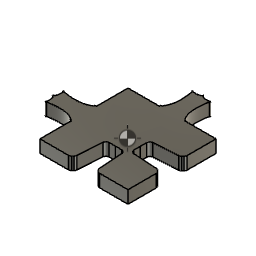
peg-design-block v3 (Autodesk Fusion 360 design; units mm, degrees)
Autodesk Fusion 360 part; units mm, degrees
note: some values were not read from the file. Set by a fixed rule: which sketch regions a step uses.
sketch "Sketch1" plane through (0, 0, 0) normal (0, 0, 1) x (1, 0, 0)
  line L0 (10, 10) -> (-10, 10)
  line L1 (0, 10) -> (0, 20)
  line L2 (-10, 10) -> (-4, 10)
  line L3 (10, 10) -> (4, 10)
  line L4 (0, 20) -> (0, 19.3)
  line L5 (0, 20) -> (0, 19.9)
  line L6 (-3, 11) -> (-2.5, 11)
  line L7 (3, 11) -> (2.5, 11)
  line L8 (-10, 10) -> (-11, 10)
  line L9 (11, 10) -> (10, 10)
  line L10 (0, 10) -> (-4.5, 10)
  line L11 (0, 10) -> (4.5, 10)
  line L12 (0, 10) -> (0, 20)
  line L13 (4, 10.5) -> (4, 10.4)
  line L14 (4, 10.5) -> (4, 10.4)
  line L15 (-2.5, 11) -> (-2.5, 13.5)
  line L16 (2.5, 11) -> (2.5, 13.5)
  line L17 (-4, 10) -> (-3.8, 10)
  line L18 (-4, 10) -> (-3.8, 10.3)
  circle A0 centre (-3.8, 10.3) radius 0.2
  circle A1 centre (3.8, 10.3) radius 0.2
  line L19 (3.8, 10.3) -> (4, 10)
  line L20 (0, 20) -> (0, 19.4)
  line L21 (0, 20) -> (0, 19.3)
  circle A2 centre (2.8, 19.3) radius 0.2
  circle A3 centre (-2.8, 19.3) radius 0.2
  line L22 (0, 20) -> (0, 19.8)
  circle A4 centre (0, 19.8) radius 0.2
  spline S0 degree 5 poles (0, 19.8) (-0.0322, 19.7692) (-0.0986, 19.7096) (-0.2048, 19.6258) (-0.3594, 19.5254) (-0.576, 19.4201) (-0.8177, 19.3367) (-1.0861, 19.2766) (-1.3815, 19.2401) (-1.7022, 19.2255) (-2.046, 19.2311) (-2.3378, 19.2501) (-2.5655, 19.2721) (-2.7212, 19.2901) (-2.8, 19.3) knots 0 0 0 0 0 0 0.1 0.2 0.3 0.4 0.5 0.6 0.7 0.8 0.9 1 1 1 1 1 1
  spline S1 degree 5 poles (0, 19.8) (0.0322, 19.7692) (0.0986, 19.7096) (0.2048, 19.6258) (0.3594, 19.5254) (0.576, 19.4201) (0.8177, 19.3367) (1.0861, 19.2766) (1.3815, 19.2401) (1.7022, 19.2255) (2.046, 19.2311) (2.3378, 19.2501) (2.5655, 19.2721) (2.7212, 19.2901) (2.8, 19.3) knots 0 0 0 0 0 0 0.1 0.2 0.3 0.4 0.5 0.6 0.7 0.8 0.9 1 1 1 1 1 1
  spline S2 degree 5 poles (-2.8, 19.3) (-2.7571, 19.0585) (-2.6765, 18.5805) (-2.5713, 17.879) (-2.4629, 16.9749) (-2.3846, 15.9005) (-2.3693, 14.8878) (-2.4235, 13.943) (-2.5527, 13.0716) (-2.7578, 12.2743) (-3.0346, 11.5472) (-3.3095, 11.0177) (-3.5439, 10.6483) (-3.7126, 10.4141) (-3.8, 10.3) knots 0 0 0 0 0 0 0.1 0.2 0.3 0.4 0.5 0.6 0.7 0.8 0.9 1 1 1 1 1 1
  spline S3 degree 5 poles (2.8, 19.3) (2.7571, 19.0585) (2.6765, 18.5805) (2.5713, 17.879) (2.4629, 16.9749) (2.3846, 15.9005) (2.3693, 14.8878) (2.4235, 13.943) (2.5527, 13.0716) (2.7578, 12.2743) (3.0346, 11.5472) (3.3095, 11.0177) (3.5439, 10.6483) (3.7126, 10.4141) (3.8, 10.3) knots 0 0 0 0 0 0 0.1 0.2 0.3 0.4 0.5 0.6 0.7 0.8 0.9 1 1 1 1 1 1
  line L23 (-2.8, 19.3) -> (-2.8, 19.5)
  line L24 (-2.8, 19.5) -> (-3, 19.5)
  line L25 (0, 20) -> (0, 19.8)
  line L26 (0, 20) -> (0, 19.3)
  line L27 (0, 20) -> (0, 19.9)
  circle A5 centre (0, 19.8) radius 0.2
  line L28 (0, 10) -> (0, 20)
  line L29 (4, 10.5) -> (4, 10.4)
  line L30 (0, 10) -> (0, 20)
  line L31 (4, 10.5) -> (4, 10.4)
  circle A6 centre (3.8, 10.3) radius 0.2
  line L32 (-4, 10) -> (-3.8, 10)
  line L33 (3.8, 10.3) -> (4, 10)
  line L34 (3, 11) -> (2.5, 11)
  line L35 (-3, 11) -> (-2.5, 11)
  circle A7 centre (-3.8, 10.3) radius 0.2
  line L36 (-4, 10) -> (-3.8, 10.3)
  line L37 (4, 10) -> (4, 10.5)
  circle A8 centre (-2.8, 19.3) radius 0.2
  line L38 (-2.8, 19.5) -> (-3, 19.5)
  line L39 (2.5, 11) -> (2.5, 13.5)
  line L40 (0, 10) -> (-4.5, 10)
  line L41 (-2.5, 11) -> (-2.5, 13.5)
  line L42 (0, 20) -> (0, 19.3)
  spline S4 degree 5 poles (-2.8, 19.3) (-2.7571, 19.0585) (-2.6765, 18.5805) (-2.5713, 17.879) (-2.4629, 16.9749) (-2.3846, 15.9005) (-2.3693, 14.8878) (-2.4235, 13.943) (-2.5527, 13.0716) (-2.7578, 12.2743) (-3.0346, 11.5472) (-3.3095, 11.0177) (-3.5439, 10.6483) (-3.7126, 10.4141) (-3.8, 10.3) knots 0 0 0 0 0 0 0.1 0.2 0.3 0.4 0.5 0.6 0.7 0.8 0.9 1 1 1 1 1 1
  line L43 (0, 20) -> (0, 19.4)
  spline S5 degree 5 poles (0, 19.8) (-0.0322, 19.7692) (-0.0986, 19.7096) (-0.2048, 19.6258) (-0.3594, 19.5254) (-0.576, 19.4201) (-0.8177, 19.3367) (-1.0861, 19.2766) (-1.3815, 19.2401) (-1.7022, 19.2255) (-2.046, 19.2311) (-2.3378, 19.2501) (-2.5655, 19.2721) (-2.7212, 19.2901) (-2.8, 19.3) knots 0 0 0 0 0 0 0.1 0.2 0.3 0.4 0.5 0.6 0.7 0.8 0.9 1 1 1 1 1 1
  circle A9 centre (2.8, 19.3) radius 0.2
  spline S6 degree 5 poles (0, 19.8) (0.0322, 19.7692) (0.0986, 19.7096) (0.2048, 19.6258) (0.3594, 19.5254) (0.576, 19.4201) (0.8177, 19.3367) (1.0861, 19.2766) (1.3815, 19.2401) (1.7022, 19.2255) (2.046, 19.2311) (2.3378, 19.2501) (2.5655, 19.2721) (2.7212, 19.2901) (2.8, 19.3) knots 0 0 0 0 0 0 0.1 0.2 0.3 0.4 0.5 0.6 0.7 0.8 0.9 1 1 1 1 1 1
  line L44 (-2.8, 19.3) -> (-2.8, 19.5)
  spline S7 degree 5 poles (2.8, 19.3) (2.7571, 19.0585) (2.6765, 18.5805) (2.5713, 17.879) (2.4629, 16.9749) (2.3846, 15.9005) (2.3693, 14.8878) (2.4235, 13.943) (2.5527, 13.0716) (2.7578, 12.2743) (3.0346, 11.5472) (3.3095, 11.0177) (3.5439, 10.6483) (3.7126, 10.4141) (3.8, 10.3) knots 0 0 0 0 0 0 0.1 0.2 0.3 0.4 0.5 0.6 0.7 0.8 0.9 1 1 1 1 1 1
  line L45 (0, 20) -> (0, 19.8)
  line L46 (0, 20) -> (0, 19.3)
  line L47 (0, 20) -> (0, 19.9)
  circle A10 centre (0, 19.8) radius 0.2
  line L48 (0, 10) -> (0, 20)
  line L49 (4, 10.5) -> (4, 10.4)
  line L50 (0, 10) -> (0, 20)
  line L51 (4, 10.5) -> (4, 10.4)
  circle A11 centre (3.8, 10.3) radius 0.2
  line L52 (-4, 10) -> (-3.8, 10)
  line L53 (3.8, 10.3) -> (4, 10)
  line L54 (3, 11) -> (2.5, 11)
  line L55 (-3, 11) -> (-2.5, 11)
  circle A12 centre (-3.8, 10.3) radius 0.2
  line L56 (-4, 10) -> (-3.8, 10.3)
  circle A13 centre (-2.8, 19.3) radius 0.2
  line L57 (-2.8, 19.5) -> (-3, 19.5)
  line L58 (2.5, 11) -> (2.5, 13.5)
  line L59 (0, 10) -> (-4.5, 10)
  line L60 (-2.5, 11) -> (-2.5, 13.5)
  line L61 (0, 20) -> (0, 19.3)
  spline S8 degree 5 poles (-2.8, 19.3) (-2.7571, 19.0585) (-2.6765, 18.5805) (-2.5713, 17.879) (-2.4629, 16.9749) (-2.3846, 15.9005) (-2.3693, 14.8878) (-2.4235, 13.943) (-2.5527, 13.0716) (-2.7578, 12.2743) (-3.0346, 11.5472) (-3.3095, 11.0177) (-3.5439, 10.6483) (-3.7126, 10.4141) (-3.8, 10.3) knots 0 0 0 0 0 0 0.1 0.2 0.3 0.4 0.5 0.6 0.7 0.8 0.9 1 1 1 1 1 1
  line L62 (0, 20) -> (0, 19.4)
  spline S9 degree 5 poles (0, 19.8) (-0.0322, 19.7692) (-0.0986, 19.7096) (-0.2048, 19.6258) (-0.3594, 19.5254) (-0.576, 19.4201) (-0.8177, 19.3367) (-1.0861, 19.2766) (-1.3815, 19.2401) (-1.7022, 19.2255) (-2.046, 19.2311) (-2.3378, 19.2501) (-2.5655, 19.2721) (-2.7212, 19.2901) (-2.8, 19.3) knots 0 0 0 0 0 0 0.1 0.2 0.3 0.4 0.5 0.6 0.7 0.8 0.9 1 1 1 1 1 1
  circle A14 centre (2.8, 19.3) radius 0.2
  spline S10 degree 5 poles (0, 19.8) (0.0322, 19.7692) (0.0986, 19.7096) (0.2048, 19.6258) (0.3594, 19.5254) (0.576, 19.4201) (0.8177, 19.3367) (1.0861, 19.2766) (1.3815, 19.2401) (1.7022, 19.2255) (2.046, 19.2311) (2.3378, 19.2501) (2.5655, 19.2721) (2.7212, 19.2901) (2.8, 19.3) knots 0 0 0 0 0 0 0.1 0.2 0.3 0.4 0.5 0.6 0.7 0.8 0.9 1 1 1 1 1 1
  line L63 (-2.8, 19.3) -> (-2.8, 19.5)
  spline S11 degree 5 poles (2.8, 19.3) (2.7571, 19.0585) (2.6765, 18.5805) (2.5713, 17.879) (2.4629, 16.9749) (2.3846, 15.9005) (2.3693, 14.8878) (2.4235, 13.943) (2.5527, 13.0716) (2.7578, 12.2743) (3.0346, 11.5472) (3.3095, 11.0177) (3.5439, 10.6483) (3.7126, 10.4141) (3.8, 10.3) knots 0 0 0 0 0 0 0.1 0.2 0.3 0.4 0.5 0.6 0.7 0.8 0.9 1 1 1 1 1 1
  line L64 (-11, 10) -> (-12, 10)
  line L65 (12, 10) -> (11, 10)
  line L66 (-12, 10) -> (-14, 10)
  line L67 (-14, 10) -> (-14, -18)
  line L68 (-14, -18) -> (14, -18)
  line L69 (14, -18) -> (14, 10)
  line L70 (14, 10) -> (12, 10)
  line L71 (-14, 10) -> (14, -18)
  line L72 (-2.9666, -8.002) -> (0, -8)
  line L73 (2.9666, -8.002) -> (0, -8)
  line L74 (-3, -8.5) -> (-2.9666, -8.002)
  line L75 (3, -8.5) -> (2.9666, -8.002)
  line L76 (-3.5757, -17.0757) -> (-3, -8.5)
  line L77 (3.5757, -17.0757) -> (3, -8.5)
  line L78 (-4, -17.5) -> (-3.5757, -17.0757)
  line L79 (4, -17.5) -> (3.5757, -17.0757)
  line L80 (-4.5, -18) -> (-4, -17.5)
  line L81 (4.5, -18) -> (4, -17.5)
  line L82 (4.002, -7.0666) -> (4, -4.1)
  line L83 (4.002, -1.1334) -> (4, -4.1)
  line L84 (4.5, -7.1) -> (4.002, -7.0666)
  line L85 (4.5, -1.1) -> (4.002, -1.1334)
  line L86 (13.0757, -7.6757) -> (4.5, -7.1)
  line L87 (13.0757, -0.5243) -> (4.5, -1.1)
  line L88 (13.5, -8.1) -> (13.0757, -7.6757)
  line L89 (13.5, -0.1) -> (13.0757, -0.5243)
  line L90 (14, -8.6) -> (13.5, -8.1)
  line L91 (14, 0.4) -> (13.5, -0.1)
  line L92 (-14.5, 0) -> (-14.4, 0)
  line L93 (-15, -1.5) -> (-17.5, -1.5)
  line L94 (-14.3, -0.2) -> (-14, 0)
  line L95 (-14.5, 0) -> (-14.4, 0)
  line L96 (-14, -4) -> (-14, -8.5)
  line L97 (-23.5, -6.8) -> (-23.5, -7)
  spline S12 degree 5 poles (-23.3, -6.8) (-23.0585, -6.7571) (-22.5805, -6.6765) (-21.879, -6.5713) (-20.9749, -6.4629) (-19.9005, -6.3846) (-18.8878, -6.3693) (-17.943, -6.4235) (-17.0716, -6.5527) (-16.2743, -6.7578) (-15.5472, -7.0346) (-15.0177, -7.3095) (-14.6483, -7.5439) (-14.4141, -7.7126) (-14.3, -7.8) knots 0 0 0 0 0 0 0.1 0.2 0.3 0.4 0.5 0.6 0.7 0.8 0.9 1 1 1 1 1 1
  spline S13 degree 5 poles (-23.3, -6.8) (-23.0585, -6.7571) (-22.5805, -6.6765) (-21.879, -6.5713) (-20.9749, -6.4629) (-19.9005, -6.3846) (-18.8878, -6.3693) (-17.943, -6.4235) (-17.0716, -6.5527) (-16.2743, -6.7578) (-15.5472, -7.0346) (-15.0177, -7.3095) (-14.6483, -7.5439) (-14.4141, -7.7126) (-14.3, -7.8) knots 0 0 0 0 0 0 0.1 0.2 0.3 0.4 0.5 0.6 0.7 0.8 0.9 1 1 1 1 1 1
  spline S14 degree 5 poles (-23.3, -1.2) (-23.0585, -1.2429) (-22.5805, -1.3235) (-21.879, -1.4287) (-20.9749, -1.5371) (-19.9005, -1.6154) (-18.8878, -1.6307) (-17.943, -1.5765) (-17.0716, -1.4473) (-16.2743, -1.2422) (-15.5472, -0.9654) (-15.0177, -0.6905) (-14.6483, -0.4561) (-14.4141, -0.2874) (-14.3, -0.2) knots 0 0 0 0 0 0 0.1 0.2 0.3 0.4 0.5 0.6 0.7 0.8 0.9 1 1 1 1 1 1
  spline S15 degree 5 poles (-23.3, -1.2) (-23.0585, -1.2429) (-22.5805, -1.3235) (-21.879, -1.4287) (-20.9749, -1.5371) (-19.9005, -1.6154) (-18.8878, -1.6307) (-17.943, -1.5765) (-17.0716, -1.4473) (-16.2743, -1.2422) (-15.5472, -0.9654) (-15.0177, -0.6905) (-14.6483, -0.4561) (-14.4141, -0.2874) (-14.3, -0.2) knots 0 0 0 0 0 0 0.1 0.2 0.3 0.4 0.5 0.6 0.7 0.8 0.9 1 1 1 1 1 1
  spline S16 degree 5 poles (-23.3, -1.2) (-23.0585, -1.2429) (-22.5805, -1.3235) (-21.879, -1.4287) (-20.9749, -1.5371) (-19.9005, -1.6154) (-18.8878, -1.6307) (-17.943, -1.5765) (-17.0716, -1.4473) (-16.2743, -1.2422) (-15.5472, -0.9654) (-15.0177, -0.6905) (-14.6483, -0.4561) (-14.4141, -0.2874) (-14.3, -0.2) knots 0 0 0 0 0 0 0.1 0.2 0.3 0.4 0.5 0.6 0.7 0.8 0.9 1 1 1 1 1 1
  line L98 (-14, -4) -> (-24, -4)
  spline S17 degree 5 poles (-23.8, -4) (-23.7692, -4.0322) (-23.7096, -4.0986) (-23.6258, -4.2048) (-23.5254, -4.3594) (-23.4201, -4.576) (-23.3367, -4.8177) (-23.2766, -5.0861) (-23.2401, -5.3815) (-23.2255, -5.7022) (-23.2311, -6.046) (-23.2501, -6.3378) (-23.2721, -6.5655) (-23.2901, -6.7212) (-23.3, -6.8) knots 0 0 0 0 0 0 0.1 0.2 0.3 0.4 0.5 0.6 0.7 0.8 0.9 1 1 1 1 1 1
  spline S18 degree 5 poles (-23.8, -4) (-23.7692, -4.0322) (-23.7096, -4.0986) (-23.6258, -4.2048) (-23.5254, -4.3594) (-23.4201, -4.576) (-23.3367, -4.8177) (-23.2766, -5.0861) (-23.2401, -5.3815) (-23.2255, -5.7022) (-23.2311, -6.046) (-23.2501, -6.3378) (-23.2721, -6.5655) (-23.2901, -6.7212) (-23.3, -6.8) knots 0 0 0 0 0 0 0.1 0.2 0.3 0.4 0.5 0.6 0.7 0.8 0.9 1 1 1 1 1 1
  line L99 (-14, -8) -> (-14.3, -7.8)
  spline S19 degree 5 poles (-23.8, -4) (-23.7692, -3.9678) (-23.7096, -3.9014) (-23.6258, -3.7952) (-23.5254, -3.6406) (-23.4201, -3.424) (-23.3367, -3.1823) (-23.2766, -2.9139) (-23.2401, -2.6185) (-23.2255, -2.2978) (-23.2311, -1.954) (-23.2501, -1.6622) (-23.2721, -1.4345) (-23.2901, -1.2788) (-23.3, -1.2) knots 0 0 0 0 0 0 0.1 0.2 0.3 0.4 0.5 0.6 0.7 0.8 0.9 1 1 1 1 1 1
  spline S20 degree 5 poles (-23.8, -4) (-23.7692, -3.9678) (-23.7096, -3.9014) (-23.6258, -3.7952) (-23.5254, -3.6406) (-23.4201, -3.424) (-23.3367, -3.1823) (-23.2766, -2.9139) (-23.2401, -2.6185) (-23.2255, -2.2978) (-23.2311, -1.954) (-23.2501, -1.6622) (-23.2721, -1.4345) (-23.2901, -1.2788) (-23.3, -1.2) knots 0 0 0 0 0 0 0.1 0.2 0.3 0.4 0.5 0.6 0.7 0.8 0.9 1 1 1 1 1 1
  spline S21 degree 5 poles (-23.8, -4) (-23.7692, -3.9678) (-23.7096, -3.9014) (-23.6258, -3.7952) (-23.5254, -3.6406) (-23.4201, -3.424) (-23.3367, -3.1823) (-23.2766, -2.9139) (-23.2401, -2.6185) (-23.2255, -2.2978) (-23.2311, -1.954) (-23.2501, -1.6622) (-23.2721, -1.4345) (-23.2901, -1.2788) (-23.3, -1.2) knots 0 0 0 0 0 0 0.1 0.2 0.3 0.4 0.5 0.6 0.7 0.8 0.9 1 1 1 1 1 1
  circle A15 centre (-23.3, -1.2) radius 0.2
  circle A16 centre (-23.3, -1.2) radius 0.2
  spline S22 degree 5 poles (-23.8, -4) (-23.7692, -4.0322) (-23.7096, -4.0986) (-23.6258, -4.2048) (-23.5254, -4.3594) (-23.4201, -4.576) (-23.3367, -4.8177) (-23.2766, -5.0861) (-23.2401, -5.3815) (-23.2255, -5.7022) (-23.2311, -6.046) (-23.2501, -6.3378) (-23.2721, -6.5655) (-23.2901, -6.7212) (-23.3, -6.8) knots 0 0 0 0 0 0 0.1 0.2 0.3 0.4 0.5 0.6 0.7 0.8 0.9 1 1 1 1 1 1
  circle A17 centre (-23.8, -4) radius 0.2
  line L100 (-23.3, -6.8) -> (-23.5, -6.8)
  spline S23 degree 5 poles (-23.3, -6.8) (-23.0585, -6.7571) (-22.5805, -6.6765) (-21.879, -6.5713) (-20.9749, -6.4629) (-19.9005, -6.3846) (-18.8878, -6.3693) (-17.943, -6.4235) (-17.0716, -6.5527) (-16.2743, -6.7578) (-15.5472, -7.0346) (-15.0177, -7.3095) (-14.6483, -7.5439) (-14.4141, -7.7126) (-14.3, -7.8) knots 0 0 0 0 0 0 0.1 0.2 0.3 0.4 0.5 0.6 0.7 0.8 0.9 1 1 1 1 1 1
  line L101 (-24, -4) -> (-23.3, -4)
  circle A18 centre (-14.3, -0.2) radius 0.2
  circle A19 centre (-14.3, -0.2) radius 0.2
  circle A20 centre (-14.3, -0.2) radius 0.2
  line L102 (-15, -1) -> (-15, -1.5)
  line L103 (-24, -4) -> (-23.3, -4)
  line L104 (-24, -4) -> (-23.4, -4)
  circle A21 centre (-23.8, -4) radius 0.2
  circle A22 centre (-23.3, -6.8) radius 0.2
  line L105 (-24, -4) -> (-23.4, -4)
  line L106 (-23.5, -6.8) -> (-23.5, -7)
  line L107 (-23.3, -6.8) -> (-23.5, -6.8)
  circle A23 centre (-23.8, -4) radius 0.2
  line L108 (-24, -4) -> (-23.3, -4)
  line L109 (-23.5, -6.8) -> (-23.5, -7)
  line L110 (-24, -4) -> (-23.8, -4)
  line L111 (-23.3, -6.8) -> (-23.5, -6.8)
  circle A24 centre (-23.3, -6.8) radius 0.2
  line L112 (-24, -4) -> (-23.4, -4)
  line L113 (-24, -4) -> (-23.3, -4)
  line L114 (-24, -4) -> (-23.8, -4)
  circle A25 centre (-23.3, -6.8) radius 0.2
  line L115 (-24, -4) -> (-23.3, -4)
  line L116 (-14, 0) -> (-14.5, 0)
  line L117 (-15, -6.5) -> (-17.5, -6.5)
  circle A26 centre (-14.3, -7.8) radius 0.2
  line L118 (-15, -6.5) -> (-17.5, -6.5)
  line L119 (-15, -7) -> (-15, -6.5)
  line L120 (-14, -4) -> (-24, -4)
  circle A27 centre (-14.3, -7.8) radius 0.2
  line L121 (-24, -4) -> (-23.3, -4)
  line L122 (-24, -4) -> (-23.9, -4)
  line L123 (-24, -4) -> (-23.8, -4)
  line L124 (-24, -4) -> (-23.9, -4)
  line L125 (-24, -4) -> (-23.9, -4)
  line L126 (-15, -1.5) -> (-17.5, -1.5)
  line L127 (-14.5, 0) -> (-14.4, 0)
  line L128 (-14.5, 0) -> (-14.4, 0)
  line L129 (-15, -1) -> (-15, -1.5)
  line L130 (-15, -1.5) -> (-17.5, -1.5)
  line L131 (-15, -1) -> (-15, -1.5)
  line L132 (-14.5, 0) -> (-14.4, 0)
  line L133 (-14, -4) -> (-24, -4)
  line L134 (-14, -8) -> (-14, -7.8)
  line L135 (-14, -4) -> (-24, -4)
  line L136 (-14, -8) -> (-14.3, -7.8)
  line L137 (-14, -4) -> (-24, -4)
  circle A28 centre (-14.3, -7.8) radius 0.2
  line L138 (-14, -8) -> (-14.3, -7.8)
  line L139 (-14, -4) -> (-14, 0.5)
  line L140 (-14, -4) -> (-14, -8.5)
  circle A29 centre (-23.3, -1.2) radius 0.2
  line L141 (-14.3, -0.2) -> (-14, 0)
  line L142 (-15, -7) -> (-15, -6.5)
  line L143 (-14.3, -0.2) -> (-14, 0)
  line L144 (-14, -4) -> (-24, -4)
  line L145 (-14, -8) -> (-14, -7.8)
  line L146 (-15, -7) -> (-15, -6.5)
  line L147 (-14, -4) -> (-14, -8.5)
  line L148 (-15, -6.5) -> (-17.5, -6.5)
  line L149 (-14, -8) -> (-14, -7.8)
  line L150 (-14.5, 0) -> (-14.4, 0)
  point P0 (-1, 19.3)
  point P1 (1, 19.3)
  point P2 (-1, 19.3)
  point P3 (1, 19.3)
  point P4 (-1, 19.3)
  point P5 (1, 19.3)
  point P6 (0, -8.1)
  point P7 (4, -4.1)
  point P8 (-23.3, -5)
  point P9 (-23.3, -3)
  point P10 (-23.3, -5)
  point P11 (-23.3, -3)
  point P12 (-23.3, -3)
  point P13 (-23.3, -5)
  dimension "d3" = 6
  dimension "d4" = 6
  dimension "d11" = 0.7
  dimension "d16" = 0.1
  dimension "d17" = 1
  dimension "d18" = 1
  dimension "d23" = 0.5
  dimension "d25" = 0.5
  dimension "d32" = 1
  dimension "d36" = 4.5
  dimension "d37" = 4.5
  dimension "d38" = 10
  dimension "d41" = 0.5
  dimension "d42" = 2.5
  dimension "d43" = 2.5
  dimension "d45" = 0.4
  dimension "d46" = 0.7
  dimension "d48" = 0.4
  dimension "d49" = 0.4
  dimension "d52" = 0.7
  dimension "d53" = 0.1
  dimension "d54" = 1
  dimension "d55" = 1
  dimension "d56" = 0.5
  dimension "d57" = 0.5
  dimension "d58" = 4.5
  dimension "d59" = 10
  dimension "d60" = 0.5
  dimension "d61" = 2.5
  dimension "d62" = 2.5
  dimension "d63" = 0.4
  dimension "d64" = 0.7
  dimension "d65" = 2.8
  dimension "d66" = 0.4
  dimension "d67" = 0.4
  dimension "d70" = 0.7
  dimension "d71" = 0.1
  dimension "d72" = 1
  dimension "d73" = 1
  dimension "d74" = 0.5
  dimension "d75" = 0.5
  dimension "d76" = 4.5
  dimension "d77" = 10
  dimension "d78" = 0.5
  dimension "d79" = 2.5
  dimension "d80" = 2.5
  dimension "d81" = 0.4
  dimension "d82" = 0.7
  dimension "d83" = 2.8
  dimension "d84" = 0.4
  dimension "d85" = 0.4
  dimension "d148" = 2
  dimension "d149" = 28
  dimension "d150" = 28
  dimension "d151" = 28
  dimension "d153" = 0.6
  dimension "d154" = 0.6
  dimension "d155" = 0.7
  dimension "d156" = 0.1
  dimension "d157" = 1
  dimension "d158" = 1
  dimension "d159" = 0.5
  dimension "d160" = 0.5
  dimension "d161" = 4.5
  dimension "d162" = 4.5
  dimension "d163" = 10
  dimension "d164" = 0.5
  dimension "d165" = 2.5
  dimension "d166" = 2.5
  dimension "d167" = 0.4
  dimension "d168" = 0.7
  dimension "d169" = 0.4
  dimension "d170" = 0.4
  dimension "d171" = 0.7
  dimension "d172" = 0.1
  dimension "d173" = 1
  dimension "d174" = 1
  dimension "d175" = 0.5
  dimension "d176" = 0.5
  dimension "d177" = 4.5
  dimension "d178" = 10
  dimension "d179" = 0.5
  dimension "d180" = 2.5
  dimension "d181" = 2.5
  dimension "d182" = 0.4
  dimension "d183" = 0.7
  dimension "d184" = 2.8
  dimension "d185" = 0.4
  dimension "d186" = 0.4
  dimension "d187" = 0.7
  dimension "d188" = 0.1
  dimension "d189" = 1
  dimension "d190" = 1
  dimension "d191" = 0.5
  dimension "d192" = 0.5
  dimension "d193" = 4.5
  dimension "d194" = 10
  dimension "d195" = 0.5
  dimension "d196" = 2.5
  dimension "d197" = 2.5
  dimension "d198" = 0.4
  dimension "d199" = 0.7
  dimension "d200" = 2.8
  dimension "d201" = 0.4
  dimension "d202" = 0.4
  constraint horizontal L0
  constraint midpoint L0 L1.start
  constraint perpendicular L0 L1
  constraint parallel L1 L4
  constraint parallel L1 L5
  constraint perpendicular L1 L10
  constraint perpendicular L1 L11
  constraint perpendicular L10 L12
  constraint perpendicular L7 L14
  constraint perpendicular L6 L15
  constraint perpendicular L7 L16
  constraint coincident L10 L17.end
  constraint parallel L10 L17
  constraint coincident L18.end A0.centre
  constraint coincident A1.centre L19.start
  constraint coincident L4 L20.end
  constraint coincident A2.centre S1.end
  constraint coincident A3.centre S0.end
  constraint coincident L21 L22.end
  constraint coincident L22.end A4.centre
  constraint coincident L1.end A4
  constraint coincident A3 L23.end
  constraint vertical L23
  constraint tangent A3 L24
  constraint parallel L26 L30
  constraint parallel L27 L30
  constraint perpendicular L30 L40
  constraint perpendicular L28 L40
  constraint perpendicular L31 L34
  constraint perpendicular L35 L41
  constraint perpendicular L34 L39
  constraint coincident L17.end L40
  constraint parallel L32 L40
  constraint coincident L20.end L26
  constraint coincident L22.end L42
  constraint coincident L1.end A5
  constraint coincident L23.end A8
  constraint vertical L44
  constraint tangent A8 L38
  constraint parallel L46 L50
  constraint parallel L47 L50
  constraint perpendicular L50 L59
  constraint perpendicular L48 L59
  constraint perpendicular L51 L54
  constraint perpendicular L55 L60
  constraint perpendicular L54 L58
  constraint coincident L17.end L59
  constraint parallel L52 L59
  constraint coincident L20.end L46
  constraint coincident L22.end L61
  constraint coincident L1.end A10
  constraint coincident L23.end A13
  constraint vertical L63
  constraint tangent A13 L57
  constraint perpendicular L66 L67
  constraint perpendicular L67 L68
  constraint perpendicular L68 L69
  constraint parallel L78 L80
  constraint parallel L74 L76
  constraint parallel L88 L90
  constraint parallel L84 L86
  constraint parallel L115 L137
  constraint parallel L124 L137
  constraint perpendicular L96 L137
  constraint perpendicular L137 L139
  constraint perpendicular L96 L144
  constraint perpendicular L129 L132
  constraint perpendicular L118 L142
  constraint perpendicular L93 L129
  constraint coincident L134.end L96
  constraint parallel L96 L134
  constraint coincident S12.end S13.end
  constraint coincident L94.start S14.end
  constraint coincident L104.end L115
  constraint coincident S14.start S15.start
  constraint coincident S12.start S13.start
  constraint coincident S17.start L103
  constraint coincident S17.start S18.start
  constraint coincident L98.end A21
  constraint coincident L97.start A24
  constraint tangent L109 A24
  constraint parallel L101 L133
  constraint parallel L125 L133
  constraint perpendicular L133 L147
  constraint perpendicular L120 L147
  constraint perpendicular L128 L131
  constraint perpendicular L117 L119
  constraint perpendicular L126 L131
  constraint coincident L134.end L147
  constraint parallel L147 L149
  constraint coincident L104.end L101
  constraint coincident S17.start L113
  constraint coincident L98.end A17
  constraint coincident L97.start A22
  constraint tangent L97 A22
  constraint parallel L98 L108
  constraint parallel L98 L122
  constraint perpendicular L98 L140
  constraint perpendicular L135 L140
  constraint perpendicular L102 L127
  constraint perpendicular L146 L148
  constraint perpendicular L102 L130
  constraint coincident L134.end L140
  constraint parallel L140 L145
  constraint coincident L104.end L108
  constraint coincident S17.start L121
  constraint coincident L98.end A23
  constraint coincident L97.start A25
  constraint tangent L106 A25
  measures "d3" distance of L0.end L2.end
  measures "d4" distance of L0.start L3.end
  measures "d11" distance of L1.end L4.end
  measures "d16" distance of L1.end L5.end
  measures "d17" distance of L4.end P4
  measures "d18" distance of L4.end P5
  measures "d23" distance of L6.start L6.end
  measures "d25" distance of L7.start L7.end
  measures "d32" distance of L0.end L8.end
  measures "d36" distance of L1.start L10.end
  measures "d37" distance of L1.start L11.end
  measures "d38" distance of L1.start L1.end
  measures "d41" distance of L3.end L13.start
  measures "d42" distance of L6.end L15.end
  measures "d43" distance of L7.end L16.end
  measures "d45" diameter of A1
  measures "d46" distance of L1.end L4.end
  measures "d48" diameter of A2
  measures "d49" diameter of A3
  measures "d52" distance of L4.end L1.end
  measures "d53" distance of L1.end L5.end
  measures "d54" distance of P4 L4.end
  measures "d55" distance of P5 L4.end
  measures "d56" distance of L6.end L6.start
  measures "d57" distance of L7.end L7.start
  measures "d58" distance of L1.start L10.end
  measures "d59" distance of L1.start L1.end
  measures "d60" distance of L3.end L13.start
  measures "d61" distance of L6.end L15.end
  measures "d62" distance of L16.end L7.end
  measures "d63" diameter of A6
  measures "d64" distance of L1.end L4.end
  measures "d65" distance of L4.end A2.centre
  measures "d66" diameter of A9
  measures "d67" diameter of A8
  measures "d70" distance of L4.end L1.end
  measures "d71" distance of L1.end L5.end
  measures "d72" distance of P4 L4.end
  measures "d73" distance of P5 L4.end
  measures "d74" distance of L6.end L6.start
  measures "d75" distance of L7.end L7.start
  measures "d76" distance of L1.start L10.end
  measures "d77" distance of L1.start L1.end
  measures "d78" distance of L3.end L13.start
  measures "d79" distance of L6.end L15.end
  measures "d80" distance of L16.end L7.end
  measures "d81" diameter of A11
  measures "d82" distance of L1.end L4.end
  measures "d83" distance of L4.end A2.centre
  measures "d84" diameter of A14
  measures "d85" diameter of A13
  measures "d148" distance of L64.end L66.end
  measures "d149" distance of L66.end L67.end
  measures "d150" distance of L67.end L68.end
  measures "d151" distance of L68.end L69.end
  measures "d153" distance of L78.start L76.start
  measures "d154" distance of L88.start L86.start
  measures "d155" distance of L101.end L98.end
  measures "d156" distance of L98.end L122.end
  measures "d157" distance of P13 L101.end
  measures "d158" distance of P12 L101.end
  measures "d159" distance of L117.start L119.start
  measures "d160" distance of L93.start L102.start
  measures "d161" distance of L96.start L96.end
  measures "d162" distance of L96.start L139.end
  measures "d163" distance of L96.start L98.end
  measures "d164" distance of L94.end L92.start
  measures "d165" distance of L117.start L117.end
  measures "d166" distance of L93.end L93.start
  measures "d167" diameter of A20
  measures "d168" distance of L98.end L101.end
  measures "d169" diameter of A16
  measures "d170" diameter of A24
  measures "d171" distance of L98.end L101.end
  measures "d172" distance of L98.end L122.end
  measures "d173" distance of L101.end P13
  measures "d174" distance of L101.end P12
  measures "d175" distance of L119.start L117.start
  measures "d176" distance of L102.start L93.start
  measures "d177" distance of L96.end L96.start
  measures "d178" distance of L98.end L96.start
  measures "d179" distance of L92.start L94.end
  measures "d180" distance of L117.end L117.start
  measures "d181" distance of L93.end L93.start
  measures "d182" diameter of A19
  measures "d183" distance of L101.end L98.end
  measures "d184" distance of S14.start L101.end
  measures "d185" diameter of A15
  measures "d186" diameter of A22
  measures "d187" distance of L101.end L98.end
  measures "d188" distance of L98.end L122.end
  measures "d189" distance of P13 L101.end
  measures "d190" distance of P12 L101.end
  measures "d191" distance of L117.start L119.start
  measures "d192" distance of L93.start L102.start
  measures "d193" distance of L96.start L96.end
  measures "d194" distance of L96.start L98.end
  measures "d195" distance of L92.start L94.end
  measures "d196" distance of L117.start L117.end
  measures "d197" distance of L93.end L93.start
  measures "d198" diameter of A18
  measures "d199" distance of L101.end L98.end
  measures "d200" distance of L101.end S14.start
  measures "d201" diameter of A29
  measures "d202" diameter of A25
extrude "Extrude1" add sketch "Sketch1" along normal blind 4 contours L0 L2 L3 L8 L9 L10 L11 L17 L32 L40 L52 L59 L64 L65 L66 L69 L70 L71 L82 L83 L84 L85 L86 L87 L88 L89 L90 L91 | L0 L1 L4 L11 L12 A1 L19 L20 L21 A2 A4 S1 S3 L26 A5 L28 L30 A6 L33 L42 L43 A9 S6 S7 L46 A10 L48 L50 A11 L53 L61 L62 A14 S10 S11 | A1 L19 A6 L33 L37 A11 L53 | L0 L1 L4 L10 L12 L17 L18 A0 L20 L21 A3 A4 S0 S2 L26 A5 L28 L30 L32 A7 L36 A8 L40 L42 S4 L43 S5 L46 A10 L48 L50 L52 A12 L56 A13 L59 L61 S8 L62 S9 | A1 L19 S3 A6 L33 S7 A11 L53 S11 | A1 L19 S3 A6 L33 S7 A11 L53 S11 | L18 A0 S2 A7 L36 S4 A12 L56 S8 | L18 A0 S2 A7 L36 S4 A12 L56 S8 | L1 L4 L12 L20 L21 A4 S0 L26 A5 L28 L30 L42 L43 S5 L46 A10 L48 L50 L61 L62 S9 | L1 L4 L12 L20 L21 A4 S1 L26 A5 L28 L30 L42 L43 S6 L46 A10 L48 L50 L61 L62 S10 | A2 S1 S3 A9 S6 S7 A14 S10 S11 | A2 S1 S3 A9 S6 S7 A14 S10 S11 | L67 L68 L71 L72 L73 L74 L75 L76 L77 L78 L79 L80 L81 L96 L134 L139 L140 L145 L147 L149 | L1 L4 L5 L12 L20 L21 L22 A4 S0 L25 L26 L27 A5 L28 L30 L42 L43 S5 L45 L46 L47 A10 L48 L50 L61 L62 S9 | L1 L4 L5 L12 L20 L21 L22 A4 S1 L25 L26 L27 A5 L28 L30 L42 L43 S6 L45 L46 L47 A10 L48 L50 L61 L62 S10 | A3 S0 L23 A8 S5 L44 A13 S9 L63 | A3 S0 S2 A8 S4 S5 A13 S8 S9 | A3 S2 L23 A8 S4 L44 A13 S8 L63 | L67 L94 S14 S15 S16 L98 S19 S20 S21 A15 A16 A17 L101 A18 A19 A20 L103 L104 A21 L105 A23 L108 L112 L113 L115 L120 L121 L133 L135 L137 L139 A29 L141 L143 L144 | L94 A18 A19 A20 L116 L141 L143 | L67 L96 S12 S13 L98 S17 S18 L99 S22 A17 S23 L101 L103 L104 A21 A22 L105 A23 L108 A24 L112 L113 A25 L115 A26 L120 A27 L121 L133 L134 L135 L136 L137 A28 L138 L140 L144 L145 L147 L149 | L94 S14 S15 S16 A18 A19 A20 L141 L143 | L94 S14 S15 S16 A18 A19 A20 L141 L143 | S12 S13 L99 S23 A26 A27 L136 A28 L138 | S12 S13 L99 S23 A26 A27 L136 A28 L138 | L98 S17 S18 S22 A17 L101 L103 L104 A21 L105 A23 L108 L112 L113 L115 L120 L121 L133 L135 L137 L144 | L98 S19 S20 S21 A17 L101 L103 L104 A21 L105 A23 L108 L112 L113 L115 L120 L121 L133 L135 L137 L144 | S14 S15 S16 S19 S20 S21 A15 A16 A29 | S14 S15 S16 S19 S20 S21 A15 A16 A29 | L98 S17 S18 S22 A17 L101 L103 L104 A21 L105 A23 L108 L110 L112 L113 L114 L115 L120 L121 L122 L123 L124 L125 L133 L135 L137 L144 | L98 S19 S20 S21 A17 L101 L103 L104 A21 L105 A23 L108 L110 L112 L113 L114 L115 L120 L121 L122 L123 L124 L125 L133 L135 L137 L144 | S12 S13 L100 S23 A22 L107 L111 A24 A25 | S12 S13 S17 S18 S22 S23 A22 A24 A25 | S17 S18 S22 L100 A22 L107 L111 A24 A25
fillet "Fillet1" radius 1 6 edges at (2.9666, -8.002, 2) (3.5757, -17.0757, 2) (4.5, -18, 2) (-4.5, -18, 2) (-3.5757, -17.0757, 2) (-2.9666, -8.002, 2)
fillet "Fillet2" radius 1 6 edges at (4.002, -1.1334, 2) (13.0757, -0.5243, 2) (14, 0.4, 2) (4.002, -7.0666, 2) (13.0757, -7.6757, 2) (14, -8.6, 2)
sketch "Sketch2" plane through (0, 0, 0) normal (0, 0, 1) x (1, 0, 0)
